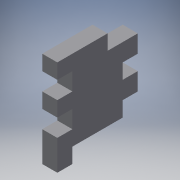
# Autodesk Inventor part: Part8
Saved by Autodesk Inventor 2018 (Build 220112000, 112)
## iProperties
Created: 2018-04-30
Part Number: Part8
Material: Generic
Document SubType Name: Modeling
Designer: Administrator
Density: 1 g/cm^3
Appearance: Default
Author: Administrator
Autodesk Inventor part; units mm, degrees
ref_plane "YZ Plane" through (0, 0, 0) normal (1, 0, 0) x (0, 1, 0)
ref_plane "XZ Plane" through (0, 0, 0) normal (0, 1, 0) x (-1, 0, 0)
ref_plane "XY Plane" through (0, 0, 0) normal (0, 0, 1) x (1, 0, 0)
sketch "Sketch1" plane through (0, 0, 0) normal (0, 1, 0) x (-1, 0, 0)
  line L0 (0, 36.314) -> (4.7625, 36.314)
  line L1 (4.7625, 36.314) -> (4.7625, 10.914)
  line L2 (4.7625, 10.914) -> (0, 10.914)
  line L3 (0, 10.914) -> (0, 36.314)
  point P0 (0, 0)
  dimension "d0" = 4.7625
  dimension "d1" = 25.4
  constraints: 8 end point, 2 parallel, 1 horizontal, 1 perpendicular
  measures "d0" distance between parallel lines of L1 L3
  measures "d1" distance between parallel lines of L2 L0
extrude "Extrusion1" add sketch "Sketch1" along normal blind 25.4
sketch "Sketch2" plane through (0, 0, 0) normal (0, -1, 0) x (1, 0, 0)
  line L0 (-4.7625, 36.314) -> (0, 36.314) projected
  line L1 (0, 36.314) -> (-4.7625, 36.314)
  line L2 (-4.7625, 36.314) -> (-4.7625, 31.5515)
  line L3 (-4.7625, 31.5515) -> (0, 31.5515)
  line L4 (0, 31.5515) -> (0, 36.314)
  point P0 (0, 0)
  dimension "d4" = 4.7625
  constraints: 8 end point, 2 parallel, 1 horizontal, 1 perpendicular
  measures "d4" distance between parallel lines of L3 L0
extrude "Extrusion2" add sketch "Sketch2" along normal blind 4.7625
sketch "Sketch4" plane through (0, 0, 10.914) normal (0, 0, -1) x (-1, 0, 0)
  line L0 (4.7625, 0) -> (4.7625, 25.4) projected
  line L1 (0, 0) -> (4.7625, 0)
  line L2 (4.7625, 0) -> (4.7625, 4.7625)
  line L3 (4.7625, 4.7625) -> (0, 4.7625)
  line L4 (0, 4.7625) -> (0, 0)
  line L5 (0, 0) -> (0, 25.4) projected
  line L6 (0, 10.3188) -> (4.7625, 10.3188)
  line L7 (4.7625, 10.3188) -> (4.7625, 15.0813)
  line L8 (4.7625, 15.0813) -> (0, 15.0813)
  line L9 (0, 15.0813) -> (0, 10.3188)
  line L10 (0, 20.6375) -> (4.7625, 20.6375)
  line L11 (4.7625, 20.6375) -> (4.7625, 25.4)
  line L12 (4.7625, 25.4) -> (0, 25.4)
  line L13 (0, 25.4) -> (0, 20.6375)
  dimension "d7" = 4.7625
  dimension "d8" = 4.7625
  dimension "d9" = 5.5563
  dimension "d10" = 5.5563
  dimension "d11" = 4.7625
  constraints: 24 end point, 6 parallel, 5 point on line, 3 horizontal, 3 perpendicular
  measures "d7" distance between parallel lines of L3 L1
  measures "d8" distance between parallel lines of L6 L8
  measures "d9" distance between parallel lines of L3 L6
  measures "d10" distance between parallel lines of L10 L8
  measures "d11" distance between parallel lines of L12 L10
extrude "Extrusion3" cut sketch "Sketch4" against normal blind 4.7625 contours L1 L4 L3 L0 | L6 L5 L8 L0 | L10 L5 L12 L0
sketch "Sketch5" plane through (-4.7625, 25.4, 36.314) normal (0, 0, 1) x (1, 0, 0)
  line L0 (4.7625, -30.1625) -> (4.7625, 0) projected
  line L1 (4.7625, -15.0812) -> (0, -15.0812)
  line L2 (0, -15.0812) -> (0, -20.6375)
  line L3 (0, -20.6375) -> (4.7625, -20.6375)
  line L4 (4.7625, -20.6375) -> (4.7625, -15.0812)
  line L5 (0, -10.3187) -> (0, -4.7625) projected
  line L6 (4.7625, -4.7625) -> (0, -4.7625)
  line L7 (0, -4.7625) -> (0, -10.3187)
  line L8 (0, -10.3187) -> (4.7625, -10.3187)
  line L9 (4.7625, -10.3187) -> (4.7625, -4.7625)
  point P0 (4.7625, -25.4)
  constraints: 16 end point, 4 parallel, 2 horizontal, 2 perpendicular, 1 midpoint, 1 point on line
extrude "Extrusion4" cut sketch "Sketch5" against normal blind 4.7625
sketch "Sketch6" plane through (0, 25.4, 0) normal (0, 1, 0) x (1, 0, 0)
  line L0 (0, -15.6765) -> (-4.7625, -15.6765) projected
  line L1 (0, -15.6765) -> (0, -31.5515) projected
  line L2 (-4.7625, -15.6765) -> (0, -15.6765)
  line L3 (0, -15.6765) -> (0, -20.439)
  line L4 (0, -20.439) -> (-4.7625, -20.439)
  line L5 (-4.7625, -20.439) -> (-4.7625, -15.6765)
  point P0 (0, 0)
  dimension "d16" = 4.7625
  constraints: 8 end point, 2 parallel, 1 horizontal, 1 perpendicular, 1 point on line
  measures "d16" distance between parallel lines of L0 L4
extrude "Extrusion5" cut sketch "Sketch6" against normal blind 4.7625
body "Solid1"
